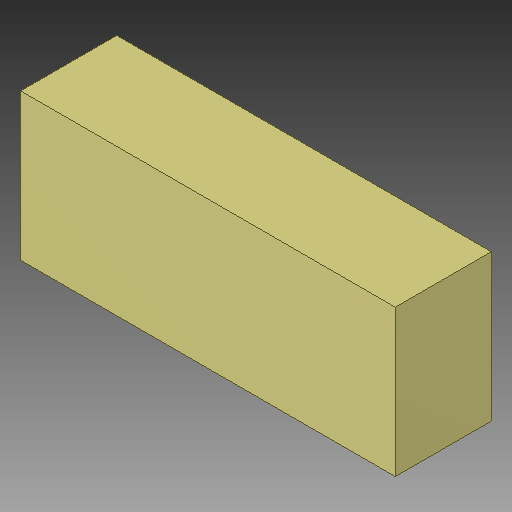
# Autodesk Inventor part: D6_SOD123
Saved by Autodesk Inventor 2017 (Build 210142000, 142)
## iProperties
Created: 2019-06-13
Part Number: D6_SOD123
Material: Generic
Document SubType Name: Modeling
Designer: Marc
Density: 1 g/cm^3
Appearance: SOD123, D6_SOD123
Author: Marc
Autodesk Inventor part; units mm, degrees
ref_plane "YZ Plane" through (0, 0, 0) normal (1, 0, 0) x (0, 1, 0)
ref_plane "XZ Plane" through (0, 0, 0) normal (0, 1, 0) x (-1, 0, 0)
ref_plane "XY Plane" through (0, 0, 0) normal (0, 0, 1) x (1, 0, 0)
sketch "SOD123, D6_SOD123_21" plane through (0, 0, 0) normal (0, 0, 1) x (1, 0, 0)
  line L0 (-1.95, 0.827) -> (1.95, 0.827)
  line L1 (1.95, 0.827) -> (1.95, -0.7)
  line L2 (1.95, -0.7) -> (-1.95, -0.7)
  line L3 (-1.95, -0.7) -> (-1.95, 0.827)
  constraints: 8 end point
extrude "Extrusion1" add sketch "SOD123, D6_SOD123_21" along normal blind 1
body "Solid1"
